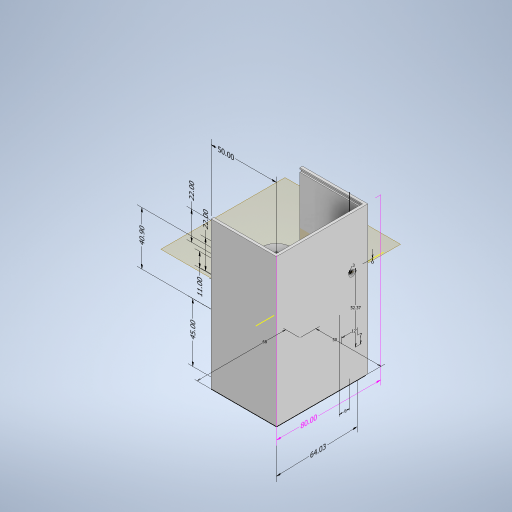
# Autodesk Inventor part: motor_maincase1.1
Saved by Autodesk Inventor 2023 (Build 270158000, 158)
## iProperties
Created: 2022-12-09
Part Number: motor_maincase1.1
Material: Generic
Document SubType Name: Modeling
Designer: jxl19
Density: 1 g/cm^3
Appearance: Default
Author: jxl19
## iProperties of the stored document motor_maincase1.1_3DPrint.ipt
Created: 2023-04-18
Part Number: motor_maincase1.1_3DPrint
Material: Generic
Document SubType Name: Modeling
Designer: jxl19
Density: 1 g/cm^3
Appearance: Default
Author: jxl19
Autodesk Inventor part; units mm, degrees
ref_plane "YZ Plane" through (0, 0, 0) normal (1, 0, 0) x (0, 1, 0)
ref_plane "XZ Plane" through (0, 0, 0) normal (0, 1, 0) x (-1, 0, 0)
ref_plane "XY Plane" through (0, 0, 0) normal (0, 0, 1) x (1, 0, 0)
sketch "Sketch1" plane through (0, 0, 0) normal (0, 1, 0) x (-1, 0, 0)
  line L0 (25, 34) -> (-25, 34)
  line L1 (-25, 34) -> (-25, -34)
  line L2 (-25, -34) -> (25, -34)
  line L3 (25, -34) -> (25, 34)
  line L4 (25, 34) -> (-25, -34) construction
  line L5 (-25, 34) -> (25, -34) construction
  point P0 (0, 0)
  dimension "d0" = 68
  dimension "d1" = 50
  constraints: 12 end point, 2 midpoint, 2 parallel, 1 horizontal, 1 perpendicular
  measures "d0" distance of L2.end L0.start
  measures "d1" distance of L1.end L2.end
extrude "left wall" add sketch "Sketch1" along normal blind 2
sketch "Sketch3" plane through (0, 2, 0) normal (0, 1, 0) x (1, 0, 0)
  line L0 (25, -34) -> (25, 34) projected
  line L1 (-25, 34) -> (-25, -34) projected
  line L2 (25, -34) -> (-25, -34)
  line L3 (-25, -34) -> (-25, -32)
  line L4 (-25, -32) -> (25, -32)
  line L5 (25, -32) -> (25, -34)
  point P0 (0, 0)
  dimension "d4" = 2
  constraints: 8 end point, 2 parallel, 1 horizontal, 1 perpendicular, 1 point on line
  measures "d4" distance of L2.end L3.end
extrude "bottom wall" add sketch "Sketch3" along normal blind 110.9
sketch "Sketch10" plane through (-25, 2, 32) normal (0, 0, -1) x (-1, 0, 0)
  line L0 (0, 0) -> (0, 110.9) projected
  line L1 (-50, 0) -> (-50, 110.9) projected
  line L2 (0, 58.9) -> (-50, 58.9)
  line L3 (-50, 58.9) -> (-50, 61.9)
  line L4 (-50, 61.9) -> (0, 61.9)
  line L5 (0, 61.9) -> (0, 58.9)
  line L6 (-50, 0) -> (0, 0) projected
  point P0 (-25, -2)
  point P1 (0, 61.9)
  point P2 (-50, 58.9)
  dimension "d33" = 3
  dimension "d34" = 58.9
  constraints: 8 end point, 2 parallel, 2 point on line, 1 horizontal, 1 perpendicular
  measures "d33" distance between parallel lines of L4 L2
  measures "d34" distance between parallel lines of L2 L6
extrude "mid wall" add sketch "Sketch10" along normal blind 48 contours L2 L1 L4 L0
sketch "Sketch11" plane through (-25, 60.9, 32) normal (0, -1, 0) x (1, 0, 0)
  circle A0 centre (24, -24) radius 2.9
  line L0 (0, 0) -> (0, -48) projected
  line L1 (0, -48) -> (50, -48) projected
  dimension "d37" = 5.8
  dimension "d136" = 24
  dimension "d137" = 24
  constraints: 1 centre point
  measures "d37" diameter of A0
  measures "d136" distance from line of L0 A0.centre
  measures "d137" distance from line of L1 A0.centre
extrude "middle bearing hole" cut sketch "Sketch11" against normal blind 48
sketch "Sketch15" plane through (0, 2, 0) normal (0, 1, 0) x (1, 0, 0)
  line L0 (25, 34) -> (-25, 34) projected
  line L1 (-25, -32) -> (25, -32) projected
  line L2 (25, 34) -> (23, 34)
  line L3 (23, 34) -> (23, -32)
  line L4 (23, -32) -> (25, -32)
  line L5 (25, -32) -> (25, 34)
  point P0 (0, 0)
  point P1 (25, -32)
  dimension "d69" = 2
  constraints: 8 end point, 2 parallel, 1 horizontal, 1 perpendicular, 1 point on line
  measures "d69" distance between parallel lines of L5 L3
extrude "back wall" add sketch "Sketch15" along normal blind 110.9
sketch "Sketch20" plane through (-25, 60.9, -16) normal (0, -1, 0) x (1, 0, 0)
  circle A0 centre (24, 24) radius 4
  line L0 (0, 48) -> (48, 48) projected
  line L1 (48, -18) -> (0, -18)
  line L2 (0, -18) -> (0, 48)
  line L3 (0, 48) -> (48, 48)
  line L4 (48, 48) -> (48, -18)
  line L5 (0, 0) -> (48, 0) projected
  point P0 (25, 16)
  point P1 (48, 48)
  point P2 (24, 0)
  dimension "d106" = 8
  dimension "d138" = 24
  dimension "d139" = 24
  constraints: 8 end point, 2 parallel, 1 centre point, 1 horizontal, 1 midpoint, 1 perpendicular
  measures "d106" diameter of A0
  measures "d138" distance of point (24, 0) A0.centre
  measures "d139" distance from line of L2 A0.centre
extrude "thicker mid wall ring for bearing" cut sketch "Sketch20" against normal blind 0.5
sketch "Sketch21" plane through (23, 2, 32) normal (0, 0, -1) x (-1, 0, 0)
  line L0 (0, 0) -> (0, 59.4) projected
  line L1 (48, -2) -> (48, 110.9) projected
  line L2 (0, 45) -> (48, 45)
  line L3 (48, 45) -> (48, 47.9)
  line L4 (48, 47.9) -> (0, 47.9)
  line L5 (0, 47.9) -> (0, 45)
  line L6 (0, 0) -> (48, 0) projected
  point P0 (23, -2)
  dimension "d110" = 45
  dimension "d111" = 2.9
  constraints: 8 end point, 2 parallel, 2 point on line, 1 horizontal, 1 perpendicular
  measures "d110" distance between parallel lines of L6 L2
  measures "d111" distance between parallel lines of L2 L4
extrude "motor attachment wall" add sketch "Sketch21" along normal up to surface (66 mm away) contours L0 L4 L1 L2
sketch "Sketch24" plane through (-25, 47, 32) normal (0, -1, 0) x (1, 0, 0)
  circle A0 centre (24, -24) radius 2.95
  circle A1 centre (20.818, -20.818) radius 0.8
  circle A2 centre (27.182, -27.182) radius 0.8
  line L0 (48, -66) -> (48, 0) projected
  line L1 (0, 0) -> (0, -66) projected
  line L2 (48, 0) -> (0, 0)
  line L3 (0, 0) -> (0, -48)
  line L4 (0, -48) -> (48, -48)
  line L5 (48, -48) -> (48, 0)
  line L6 (48, -48) -> (0, 0)
  point P0 (25, 14.5)
  dimension "d119" = 5.9
  dimension "d125" = 48
  dimension "d126" = 62.5
  dimension "d127" = 24
  dimension "d128" = 24
  dimension "d131" = 1.6
  dimension "d132" = 4.5
  dimension "d133" = 4.5
  constraints: 10 end point, 3 centre point, 3 point on line, 2 parallel, 1 horizontal, 1 midpoint, 1 perpendicular
  measures "d119" diameter of A0
  measures "d125" distance between parallel lines of L4 L2
  measures "d126" distance from line of L4 point (25, 14.5)
  measures "d127" distance from line of L4 A0.centre
  measures "d128" distance from line of L1 A0.centre
  measures "d131" diameter of A1
  measures "d132" distance of A0.centre A1.centre
  measures "d133" distance of A2.centre A0.centre
extrude "motor holes" cut sketch "Sketch24" against normal up to surface (2.9 mm away) contours A0 L6 | L6 A0 | L6 A1 | A1 L6 | L6 A2 | A2 L6
sketch "Sketch25" plane through (-25, 47, 32) normal (0, -1, 0) x (1, 0, 0)
  line L0 (48, -48) -> (0, 0)
  line L1 (0, 0) -> (0, -66) projected
  line L2 (0, 0) -> (0, -66)
  line L3 (48, -66) -> (0, -66) projected
  circle A0 centre (24, -24) radius 2.95 projected
  circle A1 centre (24, -24) radius 9
  line L4 (48, -48) -> (0, -48) projected
  line L5 (48, -48) -> (48, -66)
  line L6 (50, 2) -> (50, -66) projected
  line L7 (0, 0) -> (0, 2) projected
  line L8 (0, -66) -> (0, 0)
  point P0 (25, -32)
  point P1 (30.364, -30.364)
  point P2 (17.636, -17.636)
  dimension "d134" = 18
  constraints: 8 end point, 1 centre point, 1 coincident, 1 collinear, 1 parallel, 1 other
  measures "d134" diameter of A1
extrude "motor attachment wall cut out" cut sketch "Sketch25" against normal blind 3.075 contours L4 L1 L0 A1 | L5 L3 L1 L4
sketch "Sketch26" plane through (-25, 61.4, -16) normal (0, -1, 0) x (1, 0, 0)
  line L0 (48, 0) -> (0, 48)
  circle A0 centre (24, 24) radius 4
  circle A1 centre (24, 24) radius 2.9 projected
  line L1 (0, 0) -> (48, 0) projected
  line L2 (48, 0) -> (0, 0)
  line L3 (0, 48) -> (0, 50) projected
  line L4 (0, 0) -> (0, 48)
  line L5 (24, 24) -> (48, 24)
  line L6 (48, 48) -> (48, 0) projected
  line L7 (24, 24) -> (24, 48)
  line L8 (48, 48) -> (0, 48) projected
  line L9 (21.1716, 26.8284) -> (24, 29.6569)
  line L10 (26.8284, 21.1716) -> (29.6569, 24)
  point P0 (25, -38)
  point P1 (24, 28)
  dimension "d140" = 8
  constraints: 14 end point, 4 point on line, 2 coincident, 2 midpoint, 2 point on circle, 2 tangent, 1 centre point, 1 collinear, 1 concentric, 1 horizontal, 1 parallel, 1 perpendicular
  measures "d140" diameter of A0
extrude "mid wall cut out" cut sketch "Sketch26" against normal blind 3.075 contours L1 L4 L0 A0 | L0 L10 L5 L6 | L0 L8 L7 L9
sketch "Sketch27" plane through (23, 112.9, 32) normal (0, 0, -1) x (-1, 0, 0)
  line L0 (0, 0) -> (0, -49) projected
  line L1 (48, -112.9) -> (48, 0) projected
  line L2 (0, -27) -> (48, -27)
  line L3 (48, -27) -> (48, -25)
  line L4 (48, -25) -> (0, -25)
  line L5 (0, -25) -> (0, -27)
  line L6 (0, -110.9) -> (48, -110.9) projected
  point P0 (23, -112.9)
  point P1 (0, -25)
  dimension "d144" = 83.9
  dimension "d145" = 2
  constraints: 8 end point, 2 parallel, 2 point on line, 1 horizontal, 1 perpendicular
  measures "d144" distance between parallel lines of L6 L2
  measures "d145" distance between parallel lines of L4 L2
extrude "encoder wall" add sketch "Sketch27" along normal blind 48
sketch "Sketch28" plane through (-25, 85.9, 32) normal (0, -1, 0) x (1, 0, 0)
  line L0 (48, -48) -> (48, 0) projected
  line L1 (0, 0) -> (0, 2) projected
  line L2 (48, -48) -> (0, 0)
  circle A0 centre (24, -24) radius 3
  circle A1 centre (30.0104, -30.0104) radius 1.4
  circle A2 centre (17.9896, -17.9896) radius 1.4
  dimension "d153" = 6
  dimension "d154" = 8.5
  dimension "d155" = 8.5
  dimension "d156" = 2.8
  dimension "d157" = 2.8
  constraints: 3 centre point, 2 end point, 2 point on line, 1 coincident, 1 midpoint
  measures "d153" diameter of A0
  measures "d154" distance of A0.centre A1.centre
  measures "d155" distance of A2.centre A0.centre
  measures "d156" diameter of A1
  measures "d157" diameter of A2
extrude "encoder holes" cut sketch "Sketch28" against normal blind 48
sketch "Sketch29" plane through (-25, 85.9, 32) normal (0, -1, 0) x (1, 0, 0)
  line L0 (0, -48) -> (48, -48) projected
  line L1 (48, 0) -> (0, 0) projected
  line L2 (48, -48) -> (0, 0)
  circle A0 centre (24, -24) radius 11
  line L3 (0, 0) -> (0, 2) projected
  line L4 (0, 0) -> (0, -48)
  line L5 (0, -48) -> (48, -48)
  point P0 (25, -32)
  point P1 (31.7782, -31.7782)
  point P2 (16.2218, -16.2218)
  dimension "d160" = 22
  constraints: 6 end point, 1 centre point, 1 midpoint, 1 perpendicular, 1 vertical
  measures "d160" diameter of A0
extrude "encoder wall cut out" cut sketch "Sketch29" against normal blind 48 contours L4 L2 A0 L0
sketch "Sketch30" plane through (25, 0, -34) normal (0, 0, -1) x (-1, 0, 0)
  line L0 (2, 112.9) -> (50, 112.9) projected
  line L1 (50, 0) -> (0, 0) projected
  line L2 (50, 112.9) -> (0, 112.9)
  line L3 (0, 112.9) -> (0, 0)
  line L4 (0, 0) -> (50, 0)
  line L5 (50, 0) -> (50, 112.9)
  point P0 (25, 0)
  constraints: 8 end point, 2 parallel, 1 horizontal, 1 perpendicular
extrude "top" add sketch "Sketch30" along normal blind 2
sketch "Sketch31" plane through (25, 0, -34) normal (0, 0, 1) x (1, 0, 0)
  point P0 (-25, 0)
sketch "Sketch32" plane through (25, 0, -34) normal (0, 0, 1) x (1, 0, 0)
  line L0 (-50, 0) -> (-50, 112.9) projected
  line L1 (0, 112.9) -> (0, 0) projected
  line L2 (-50, 111.9) -> (-1, 111.9)
  line L3 (-1, 111.9) -> (-1, 109.9)
  line L4 (-1, 109.9) -> (-50, 109.9)
  line L5 (-50, 109.9) -> (-50, 111.9)
  line L6 (-50, 112.9) -> (0, 112.9) projected
  point P0 (-25, 0)
  point P1 (0, 112.9)
  dimension "d165" = 1
  dimension "d166" = 2
  dimension "d177" = 1
  constraints: 9 end point, 2 parallel, 2 perpendicular, 1 horizontal, 1 point on line
  measures "d165" distance between parallel lines of L2 L6
  measures "d166" distance between parallel lines of L4 L2
  measures "d177" distance between parallel lines of L1 L3
extrude "top rightWallGroove" cut sketch "Sketch32" against normal blind 1
sketch "Sketch33" plane through (23, 2, 32) normal (-1, 0, 0) x (0, 0, 1)
  line L0 (-78, 107.9) -> (-78, 104.9)
  line L1 (0, 110.9) -> (0, 85.9) projected
  line L2 (-78, 107.9) -> (0, 107.9)
  line L3 (0, 107.9) -> (0, 109.9)
  line L4 (0, 109.9) -> (-78, 109.9)
  line L5 (-78, 109.9) -> (-78, 107.9)
  line L6 (-66, 110.9) -> (0, 110.9) projected
  point P0 (-32, -2)
  point P1 (-78, 109.9)
  point P2 (0, 107.9)
  dimension "d169" = 2
  dimension "d178" = 1
  constraints: 10 end point, 2 parallel, 1 horizontal, 1 perpendicular, 1 point on line
  measures "d169" distance between parallel lines of L4 L2
  measures "d178" distance between parallel lines of L4 L6
extrude "back rightWallGroove" cut sketch "Sketch33" against normal blind 1
sketch "Sketch34" plane through (23, 112.9, 32) normal (0, 0, -1) x (-1, 0, 0)
  line L0 (48, -112.9) -> (48, 0) projected
  line L1 (48, -3) -> (-1, -3)
  line L2 (-1, -3) -> (-1, -1)
  line L3 (-1, -1) -> (48, -1)
  line L4 (48, -1) -> (48, -3)
  line L5 (48, 0) -> (-2, 0) projected
  line L6 (-2, -112.9) -> (-2, 0) projected
  point P0 (23, -112.9)
  point P1 (-1, -2)
  point P2 (48, -1)
  dimension "d172" = 1
  dimension "d173" = 2
  dimension "d174" = 1
  constraints: 8 end point, 2 parallel, 1 horizontal, 1 midpoint, 1 perpendicular, 1 point on line
  measures "d172" distance between parallel lines of L5 L3
  measures "d173" distance between parallel lines of L1 L3
  measures "d174" distance from line of L6 point (-1, -2)
extrude "bottom rightWallGroove" cut sketch "Sketch34" against normal blind 1
sketch "Sketch35" plane through (-25, 85.9, 32) normal (0, -1, 0) x (1, 0, 0)
  circle A0 centre (24, -24) radius 3 projected
  circle A1 centre (24, -24) radius 3
  circle A2 centre (24, -24) radius 5
  point P0 (25, -32)
  dimension "d179" = 2
  constraints: 2 centre point, 2 coincident
  measures "d179" radial gap between concentric circles of A2 A0
extrude "encoder bearing thicker" add sketch "Sketch35" along normal blind 1
ref_plane "Work Plane4" through (-1, 72.9, 32) normal (0, 1, 0) x (1, 0, 0)
sketch "Sketch38" plane through (23, 2, 32) normal (-1, 0, 0) x (0, 0, 1)
  line L0 (-66, 0) -> (-66, 107.9) projected
  line L1 (-66, 70.9) -> (-23.3371, 70.9)
  line L2 (-66, 0) -> (0, 0) projected
  line L3 (-56, 0) -> (-56, 123.7656)
  line L4 (-48, 45) -> (-48, 47.9) projected
  line L5 (-82, 70.9) -> (16, 70.9) projected
  line L6 (-62, 18.53) -> (-50, 18.53)
  line L7 (-50, 18.53) -> (-50, 25.53)
  line L8 (-50, 25.53) -> (-62, 25.53)
  line L9 (-62, 25.53) -> (-62, 18.53)
  line L10 (-62, 18.53) -> (-50, 25.53) construction
  line L11 (-50, 18.53) -> (-62, 25.53) construction
  circle A0 centre (-56, 70.9) radius 1.5
  point P0 (-32, -2)
  point P1 (-48, 46.45)
  point P2 (-56, 22.03)
  dimension "d195" = 8
  dimension "d196" = 0
  dimension "d197" = 7
  dimension "d198" = 12
  dimension "d199" = 52.37
  dimension "d202" = 3
  constraints: 16 end point, 5 point on line, 3 midpoint, 2 horizontal, 2 parallel, 1 centre point, 1 perpendicular, 1 vertical
  measures "d195" distance from line of L3 point (-48, 46.45)
  measures "d196" distance between parallel lines of L5 L1
  measures "d197" distance of L8.end L6.start
  measures "d198" distance of L7.end L8.end
  measures "d199" distance between parallel lines of L1 L6
  measures "d202" diameter of A0
extrude "loadcell block" add sketch "Sketch38" along normal blind 30 contours L6 L9 L8 L3 | L3 L8 L7 L6
extrude "wire exit" cut sketch "Sketch38" against normal blind 30 contours A0 L3 L1 | L1 L3 A0 | L3 A0 L1 | L1 A0 L3
sketch "Sketch39" plane through (-7, 2, 32) normal (-1, 0, 0) x (0, 0, 1)
  line L0 (-50, 25.53) -> (-50, 18.53) projected
  line L1 (-50, 22.03) -> (-62, 22.03)
  line L2 (-62, 25.53) -> (-62, 18.53) projected
  line L3 (-62, 18.53) -> (-50, 18.53) projected
  line L4 (-50, 18.53) -> (-62, 18.53) projected
  line L5 (-56, 18.53) -> (-56, 25.53)
  line L6 (-62, 25.53) -> (-50, 25.53) projected
  circle A0 centre (-59, 22.03) radius 1.5
  circle A1 centre (-53, 22.03) radius 1.5
  point P0 (-32, -2)
  dimension "d205" = 3.5
  dimension "d206" = 6
  dimension "d207" = 6
  dimension "d208" = 3
  dimension "d209" = 3
  constraints: 4 end point, 4 midpoint, 2 centre point, 2 point on line, 1 horizontal
  measures "d205" distance between parallel lines of L1 L3
  measures "d206" diameter of A1.centre L5
  measures "d207" diameter of A0.centre L5
  measures "d208" diameter of A0
  measures "d209" diameter of A1
extrude "loadcell screw holes" cut sketch "Sketch39" against normal blind 10 contours A1 L1 | L1 A1 | A0 L1 | L1 A0
sketch "Sketch40" plane through (23, 27.53, -18) normal (0, 1, 0) x (1, 0, 0)
  line L0 (0, -52) -> (0, 16) projected
  line L1 (0, 10) -> (-16, 10)
  line L2 (-16, 10) -> (-16, 2)
  line L3 (-16, 2) -> (0, 2)
  line L4 (0, 2) -> (0, 10)
  line L5 (-30, 0) -> (-30, 12) projected
  line L6 (0, 0) -> (-30, 0) projected
  line L7 (0, 12) -> (-30, 12) projected
  point P0 (-23, -18)
  point P1 (-16, 6)
  point P2 (-30, 6)
  point P3 (0, 2)
  dimension "d215" = 14
  dimension "d216" = 2
  dimension "d217" = 2
  constraints: 8 end point, 2 midpoint, 2 parallel, 1 horizontal, 1 perpendicular, 1 point on line
  measures "d215" distance of point (-16, 6) point (-30, 6)
  measures "d216" distance between parallel lines of L3 L6
  measures "d217" distance between parallel lines of L7 L1
extrude "Extrusion32" cut sketch "Sketch40" against normal blind 10 contours L3 L2 L1 L0
fillet "Fillet1" radius 2 4 edges at (7, 24.03, -28) (7, 24.03, -20) (23, 24.03, -20) (23, 24.03, -28)
fillet "Fillet2" radius 1 2 edges at (23, 72.9, -25.5) (25, 72.9, -25.5)
sketch "Sketch41" plane through (23, 20.53, -30) normal (0, 0, -1) x (-1, 0, 0)
  line L0 (0, 0) -> (30, 0) projected
  line L1 (0, 7) -> (30, 7) projected
  line L2 (30, 0) -> (23, 0)
  line L3 (23, 0) -> (23, 7)
  line L4 (23, 7) -> (30, 7)
  line L5 (30, 7) -> (30, 0)
  point P0 (23, -20.53)
  point P1 (23, 3.5)
  point P2 (23, 0)
  dimension "d225" = 7
  constraints: 8 end point, 2 parallel, 1 horizontal, 1 midpoint, 1 perpendicular, 1 point on line
  measures "d225" distance from line of point (23, 3.5) L5
extrude "load cell block support" add sketch "Sketch41" along normal up to surface (4 mm away)
equation "\"d136\" = d127"
equation "\"d137\" = d136"
equation "\"d69\" = d4"
equation "\"d70\" = d5"
equation "\"d138\" = d136"
equation "\"d139\" = d138"
equation "\"d127\" = 0.5 * d125"
equation "\"d128\" = d127"
equation "\"d133\" = d132"
equation "\"d134\" = 4 * d132"
equation "\"d140\" = d106"
equation "\"d146\" = d125"
equation "\"d5\" = 110.9"
body "Solid1"
